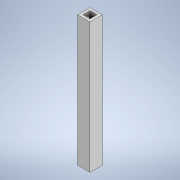
# Autodesk Inventor part: DIY composite curing oven
Saved by Autodesk Inventor 2022 (Build 260153000, 153)
## iProperties
Created: 2021-06-25
Part Number: DIY composite curing oven
Material: Generic
Document SubType Name: Modeling
Designer: Ferdinand Hubbard
Density: 1 g/cm^3
Appearance: Default
Author: Ferdinand Hubbard
Autodesk Inventor part; units mm, degrees
ref_plane "YZ Plane" through (0, 0, 0) normal (1, 0, 0) x (0, 1, 0)
ref_plane "XZ Plane" through (0, 0, 0) normal (0, 1, 0) x (-1, 0, 0)
ref_plane "XY Plane" through (0, 0, 0) normal (0, 0, 1) x (1, 0, 0)
sketch "Sketch1" plane through (0, 0, 0) normal (0, 1, 0) x (-1, 0, 0)
  line L0 (0, 0) -> (-190, 0)
  line L1 (-190, 0) -> (-190, -40)
  line L2 (-190, -40) -> (0, -40)
  line L3 (0, -40) -> (0, 0)
  line L4 (0, -40) -> (-40, -40)
  line L5 (-40, -40) -> (-40, -150)
  line L6 (-40, -150) -> (0, -150)
  line L7 (0, -150) -> (0, -40)
  line L8 (-190, -40) -> (-150, -40)
  line L9 (-150, -40) -> (-150, -150)
  line L10 (-150, -150) -> (-190, -150)
  line L11 (-190, -150) -> (-190, -40)
  line L12 (0, -150) -> (-190, -150)
  line L13 (-190, -150) -> (-190, -190)
  line L14 (-190, -190) -> (0, -190)
  line L15 (0, -190) -> (0, -150)
  circle A0 centre (-97.5466, -57.9815) radius 15.5
  circle A1 centre (-97.5466, -57.9815) radius 14
  dimension "d0" = 190
  dimension "d1" = 40
  dimension "d2" = 40
  dimension "d3" = 110
  dimension "d4" = 40
  dimension "d5" = 110
  dimension "d6" = 190
  dimension "d7" = 40
  dimension "d8" = 31
  dimension "d9" = 28
  constraints: 32 end point, 8 parallel, 4 horizontal, 4 perpendicular, 2 centre point, 1 coincident
  measures "d0" distance of L2.end L1.end
  measures "d1" distance of L1.end L0.end
  measures "d2" distance of L6.end L5.end
  measures "d3" distance of L5.end L4.end
  measures "d4" distance of L9.end L10.end
  measures "d5" distance of L8.end L9.end
  measures "d6" distance of L14.end L13.end
  measures "d7" distance of L13.end L12.end
  measures "d8" diameter of A0
  measures "d9" diameter of A1
extrude "Extrusion1" add sketch "Sketch1" along normal blind 2000 contours L3 L2 L1 L0 | L7 L6 L5 L2 | L2 L9 L10 L11 | L15 L14 L13 L10 L12 L6 | A0
body "Solid1"
